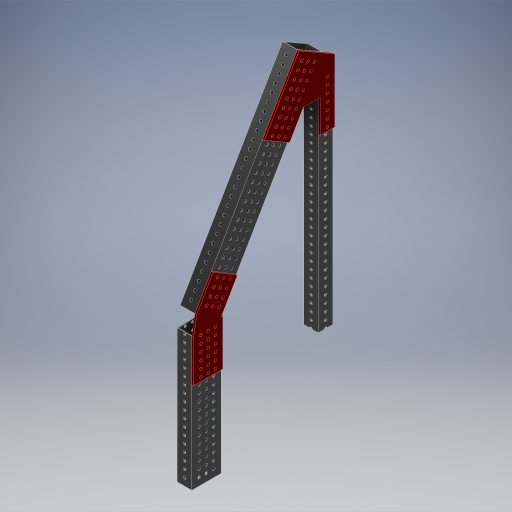
# Autodesk Inventor part: 2024-210-000-Fixed-Shootaur
Saved by Autodesk Inventor 2024.2 (Build 282272000, 272)
## iProperties
Created: 2024-01-23
Part Number: 2024-210-000-Fixed-Shootaur
Material: Generic
Document SubType Name: Modeling
Designer: rohan
Density: 1 g/cm^3
Appearance: Default
Author: rohan
Autodesk Inventor part; units mm, degrees
ref_plane "YZ Plane" through (0, 0, 0) normal (1, 0, 0) x (0, 1, 0)
ref_plane "XZ Plane" through (0, 0, 0) normal (0, 1, 0) x (-1, 0, 0)
ref_plane "XY Plane" through (0, 0, 0) normal (0, 0, 1) x (1, 0, 0)
sketch "Sketch1" plane through (0, 0, 0) normal (1, 0, 0) x (0, 1, 0)
  line L0 (47.3438, 284.2284) -> (278.9918, 284.2284)
  line L1 (278.9918, 284.2284) -> (278.9918, 233.4284)
  line L2 (278.9918, 233.4284) -> (47.3438, 233.4284)
  line L3 (618.5213, 101.1204) -> (593.1213, 57.1263)
  line L4 (593.1213, 57.1263) -> (285.1626, 234.9263)
  line L5 (285.1626, 234.9263) -> (310.5626, 278.9204)
  line L6 (310.5626, 278.9204) -> (618.5213, 101.1204)
  line L7 (285.1626, 234.9263) -> (285.1626, 48.2059)
  line L8 (310.5626, 278.9204) -> (324.8919, 270.6474)
  line L9 (47.3438, 233.4284) -> (47.3438, 284.2284)
  line L10 (47.3438, 284.2284) -> (21.9438, 284.2284)
  line L11 (21.9438, 284.2284) -> (21.9438, 233.4284)
  line L12 (21.9438, 233.4284) -> (47.3438, 233.4284)
  line L13 (47.3438, 233.4284) -> (47.3438, 284.2284)
  line L14 (21.9438, 64.4168) -> (72.7438, 64.4168)
  line L15 (72.7438, 64.4168) -> (72.7438, 39.0168)
  line L16 (72.7438, 39.0168) -> (21.9438, 39.0168)
  line L17 (21.9438, 39.0168) -> (21.9438, 64.4168)
  line L18 (21.9438, 284.2284) -> (72.7438, 284.2284)
  line L19 (72.7438, 284.2284) -> (72.7438, 724.8168)
  line L20 (72.7438, 724.8168) -> (21.9438, 724.8168)
  line L21 (21.9438, 724.8168) -> (21.9438, 284.2284)
  circle A0 centre (601.1727, 96.4718) radius 2.4892
  line L22 (72.7438, 64.4168) -> (123.5438, 64.4168)
  line L23 (123.5438, 64.4168) -> (123.5438, 39.0168)
  line L24 (123.5438, 39.0168) -> (72.7438, 39.0168)
  line L25 (72.7438, 39.0168) -> (72.7438, 64.4168)
  circle A1 centre (594.8227, 85.4733) radius 2.4892
  circle A2 centre (588.4727, 74.4748) radius 2.4892
  circle A3 centre (590.1742, 102.8218) radius 2.4892
  circle A4 centre (583.8242, 91.8233) radius 2.4892
  circle A5 centre (577.4742, 80.8248) radius 2.4892
  circle A6 centre (579.1757, 109.1718) radius 2.4892
  circle A7 centre (572.8257, 98.1733) radius 2.4892
  circle A8 centre (566.4757, 87.1748) radius 2.4892
  circle A9 centre (568.1772, 115.5218) radius 2.4892
  circle A10 centre (561.8272, 104.5233) radius 2.4892
  circle A11 centre (555.4772, 93.5248) radius 2.4892
  circle A12 centre (557.1787, 121.8718) radius 2.4892
  circle A13 centre (550.8287, 110.8733) radius 2.4892
  circle A14 centre (544.4787, 99.8748) radius 2.4892
  circle A15 centre (546.1801, 128.2218) radius 2.4892
  circle A16 centre (539.8301, 117.2233) radius 2.4892
  circle A17 centre (533.4801, 106.2248) radius 2.4892
  circle A18 centre (535.1816, 134.5718) radius 2.4892
  circle A19 centre (528.8316, 123.5733) radius 2.4892
  circle A20 centre (522.4816, 112.5748) radius 2.4892
  circle A21 centre (524.1831, 140.9218) radius 2.4892
  circle A22 centre (517.8331, 129.9233) radius 2.4892
  circle A23 centre (511.4831, 118.9248) radius 2.4892
  circle A24 centre (513.1846, 147.2718) radius 2.4892
  circle A25 centre (506.8346, 136.2733) radius 2.4892
  circle A26 centre (500.4846, 125.2748) radius 2.4892
  circle A27 centre (502.186, 153.6218) radius 2.4892
  circle A28 centre (495.836, 142.6233) radius 2.4892
  circle A29 centre (489.486, 131.6248) radius 2.4892
  circle A30 centre (491.1875, 159.9718) radius 2.4892
  circle A31 centre (484.8375, 148.9733) radius 2.4892
  circle A32 centre (478.4875, 137.9748) radius 2.4892
  circle A33 centre (480.189, 166.3218) radius 2.4892
  circle A34 centre (473.839, 155.3233) radius 2.4892
  circle A35 centre (467.489, 144.3248) radius 2.4892
  circle A36 centre (469.1905, 172.6718) radius 2.4892
  circle A37 centre (462.8405, 161.6733) radius 2.4892
  circle A38 centre (456.4905, 150.6748) radius 2.4892
  circle A39 centre (458.1919, 179.0218) radius 2.4892
  circle A40 centre (451.8419, 168.0233) radius 2.4892
  circle A41 centre (445.4919, 157.0248) radius 2.4892
  circle A42 centre (447.1934, 185.3718) radius 2.4892
  circle A43 centre (440.8434, 174.3733) radius 2.4892
  circle A44 centre (434.4934, 163.3748) radius 2.4892
  circle A45 centre (436.1949, 191.7218) radius 2.4892
  circle A46 centre (429.8449, 180.7233) radius 2.4892
  circle A47 centre (423.4949, 169.7248) radius 2.4892
  circle A48 centre (425.1964, 198.0718) radius 2.4892
  circle A49 centre (418.8464, 187.0733) radius 2.4892
  circle A50 centre (412.4964, 176.0748) radius 2.4892
  circle A51 centre (414.1979, 204.4218) radius 2.4892
  circle A52 centre (407.8479, 193.4233) radius 2.4892
  circle A53 centre (401.4979, 182.4248) radius 2.4892
  circle A54 centre (403.1993, 210.7718) radius 2.4892
  circle A55 centre (396.8493, 199.7733) radius 2.4892
  circle A56 centre (390.4993, 188.7748) radius 2.4892
  circle A57 centre (392.2008, 217.1218) radius 2.4892
  circle A58 centre (385.8508, 206.1233) radius 2.4892
  circle A59 centre (379.5008, 195.1248) radius 2.4892
  circle A60 centre (381.2023, 223.4718) radius 2.4892
  circle A61 centre (374.8523, 212.4733) radius 2.4892
  circle A62 centre (368.5023, 201.4748) radius 2.4892
  circle A63 centre (370.2038, 229.8218) radius 2.4892
  circle A64 centre (363.8538, 218.8233) radius 2.4892
  circle A65 centre (357.5038, 207.8248) radius 2.4892
  circle A66 centre (359.2052, 236.1718) radius 2.4892
  circle A67 centre (352.8552, 225.1733) radius 2.4892
  circle A68 centre (346.5052, 214.1748) radius 2.4892
  circle A69 centre (348.2067, 242.5218) radius 2.4892
  circle A70 centre (341.8567, 231.5233) radius 2.4892
  circle A71 centre (335.5067, 220.5248) radius 2.4892
  circle A72 centre (337.2082, 248.8718) radius 2.4892
  circle A73 centre (330.8582, 237.8733) radius 2.4892
  circle A74 centre (324.5082, 226.8748) radius 2.4892
  circle A75 centre (326.2097, 255.2218) radius 2.4892
  circle A76 centre (319.8597, 244.2233) radius 2.4892
  circle A77 centre (313.5097, 233.2248) radius 2.4892
  circle A78 centre (315.2112, 261.5718) radius 2.4892
  circle A79 centre (308.8612, 250.5733) radius 2.4892
  circle A80 centre (302.5112, 239.5748) radius 2.4892
  line L26 (123.5438, 64.4168) -> (568.0438, 64.4168)
  line L27 (568.0438, 64.4168) -> (568.0438, 39.0168)
  line L28 (568.0438, 39.0168) -> (123.5438, 39.0168)
  line L29 (123.5438, 39.0168) -> (123.5438, 64.4168)
  circle A81 centre (60.0438, 271.5284) radius 2.4892
  circle A82 centre (60.0438, 258.8284) radius 2.4892
  circle A83 centre (60.0438, 246.1284) radius 2.4892
  circle A84 centre (72.7438, 271.5284) radius 2.4892
  circle A85 centre (72.7438, 258.8284) radius 2.4892
  circle A86 centre (72.7438, 246.1284) radius 2.4892
  circle A87 centre (85.4438, 271.5284) radius 2.4892
  circle A88 centre (85.4438, 258.8284) radius 2.4892
  circle A89 centre (85.4438, 246.1284) radius 2.4892
  circle A90 centre (98.1438, 271.5284) radius 2.4892
  circle A91 centre (98.1438, 258.8284) radius 2.4892
  circle A92 centre (98.1438, 246.1284) radius 2.4892
  circle A93 centre (110.8438, 271.5284) radius 2.4892
  circle A94 centre (110.8438, 258.8284) radius 2.4892
  circle A95 centre (110.8438, 246.1284) radius 2.4892
  circle A96 centre (123.5438, 271.5284) radius 2.4892
  circle A97 centre (123.5438, 258.8284) radius 2.4892
  circle A98 centre (123.5438, 246.1284) radius 2.4892
  circle A99 centre (136.2438, 271.5284) radius 2.4892
  circle A100 centre (136.2438, 258.8284) radius 2.4892
  circle A101 centre (136.2438, 246.1284) radius 2.4892
  circle A102 centre (148.9438, 271.5284) radius 2.4892
  circle A103 centre (148.9438, 258.8284) radius 2.4892
  circle A104 centre (148.9438, 246.1284) radius 2.4892
  circle A105 centre (161.6438, 271.5284) radius 2.4892
  circle A106 centre (161.6438, 258.8284) radius 2.4892
  circle A107 centre (161.6438, 246.1284) radius 2.4892
  circle A108 centre (174.3438, 271.5284) radius 2.4892
  circle A109 centre (174.3438, 258.8284) radius 2.4892
  circle A110 centre (174.3438, 246.1284) radius 2.4892
  circle A111 centre (187.0438, 271.5284) radius 2.4892
  circle A112 centre (187.0438, 258.8284) radius 2.4892
  circle A113 centre (187.0438, 246.1284) radius 2.4892
  circle A114 centre (199.7438, 271.5284) radius 2.4892
  circle A115 centre (199.7438, 258.8284) radius 2.4892
  circle A116 centre (199.7438, 246.1284) radius 2.4892
  circle A117 centre (212.4438, 271.5284) radius 2.4892
  circle A118 centre (212.4438, 258.8284) radius 2.4892
  circle A119 centre (212.4438, 246.1284) radius 2.4892
  circle A120 centre (225.1438, 271.5284) radius 2.4892
  circle A121 centre (225.1438, 258.8284) radius 2.4892
  circle A122 centre (225.1438, 246.1284) radius 2.4892
  circle A123 centre (237.8438, 271.5284) radius 2.4892
  circle A124 centre (237.8438, 258.8284) radius 2.4892
  circle A125 centre (237.8438, 246.1284) radius 2.4892
  circle A126 centre (250.5438, 271.5284) radius 2.4892
  circle A127 centre (250.5438, 258.8284) radius 2.4892
  circle A128 centre (250.5438, 246.1284) radius 2.4892
  circle A129 centre (263.2438, 271.5284) radius 2.4892
  circle A130 centre (263.2438, 258.8284) radius 2.4892
  circle A131 centre (263.2438, 246.1284) radius 2.4892
  circle A132 centre (275.9438, 271.5284) radius 2.4892
  circle A133 centre (275.9438, 258.8284) radius 2.4892
  circle A134 centre (275.9438, 246.1284) radius 2.4892
  circle A135 centre (136.2438, 51.7168) radius 2.4892
  circle A136 centre (148.9438, 51.7168) radius 2.4892
  circle A137 centre (161.6438, 51.7168) radius 2.4892
  circle A138 centre (174.3438, 51.7168) radius 2.4892
  circle A139 centre (187.0438, 51.7168) radius 2.4892
  circle A140 centre (199.7438, 51.7168) radius 2.4892
  circle A141 centre (212.4438, 51.7168) radius 2.4892
  circle A142 centre (225.1438, 51.7168) radius 2.4892
  circle A143 centre (237.8438, 51.7168) radius 2.4892
  circle A144 centre (250.5438, 51.7168) radius 2.4892
  circle A145 centre (263.2438, 51.7168) radius 2.4892
  circle A146 centre (275.9438, 51.7168) radius 2.4892
  circle A147 centre (288.6438, 51.7168) radius 2.4892
  circle A148 centre (301.3438, 51.7168) radius 2.4892
  circle A149 centre (314.0438, 51.7168) radius 2.4892
  circle A150 centre (326.7438, 51.7168) radius 2.4892
  circle A151 centre (339.4438, 51.7168) radius 2.4892
  circle A152 centre (352.1438, 51.7168) radius 2.4892
  circle A153 centre (364.8438, 51.7168) radius 2.4892
  circle A154 centre (377.5438, 51.7168) radius 2.4892
  circle A155 centre (390.2438, 51.7168) radius 2.4892
  circle A156 centre (402.9438, 51.7168) radius 2.4892
  circle A157 centre (415.6438, 51.7168) radius 2.4892
  circle A158 centre (428.3438, 51.7168) radius 2.4892
  circle A159 centre (441.0438, 51.7168) radius 2.4892
  circle A160 centre (453.7438, 51.7168) radius 2.4892
  circle A161 centre (466.4438, 51.7168) radius 2.4892
  circle A162 centre (479.1438, 51.7168) radius 2.4892
  circle A163 centre (491.8438, 51.7168) radius 2.4892
  circle A164 centre (504.5438, 51.7168) radius 2.4892
  circle A165 centre (517.2438, 51.7168) radius 2.4892
  circle A166 centre (529.9438, 51.7168) radius 2.4892
  circle A167 centre (542.6438, 51.7168) radius 2.4892
  circle A168 centre (555.3438, 51.7168) radius 2.4892
  circle A169 centre (568.0438, 51.7168) radius 2.4892
  point P0 (72.7438, 51.7168)
  point P1 (568.0438, 49.2276)
  point P2 (568.0438, 54.206)
  dimension "d25" = 231.648
  dimension "d26" = 50.8
  dimension "d29" = 50.8
  dimension "d34" = 6.35
  dimension "d37" = 355.6
  dimension "d39" = 60
  dimension "d41" = 25.4
  dimension "d42" = 50.8
  dimension "d43" = 25.4
  dimension "d44" = 169.0116
  dimension "d45" = 50.8
  dimension "d46" = 440.5884
  dimension "d48" = 4.9784
  dimension "d59" = 50.8
  dimension "d60" = 12.7
  dimension "d61" = 12.7
  dimension "d64" = 12.7
  dimension "d67" = 12.7
  dimension "d70" = 444.5
  dimension "d87" = 4.9784
  dimension "d88" = 12.7
  dimension "d89" = 12.7
  dimension "d92" = 12.7
  dimension "d95" = 12.7
  dimension "d104" = 4.9784
  dimension "d105" = 12.7
  dimension "d106" = 12.7
  dimension "d109" = 12.7
  constraints: 170 centre point, 60 end point, 13 parallel, 8 horizontal, 8 perpendicular, 2 point on line, 2 vertical, 1 midpoint, 336 other
  measures "d25" distance of L1.end L2.end
  measures "d26" distance of L0.end L1.end
  measures "d29" distance of L3.start L3.end
  measures "d34" distance of L4.end L1.end
  measures "d37" distance between parallel lines of L5 L3
  measures "d39" angle of L4 L7
  measures "d41" distance of L12.end L11.end
  measures "d42" distance of L15.end L16.end
  measures "d43" distance of L14.end L15.end
  measures "d44" distance of L14.start L11.end
  measures "d45" distance of L20.end L19.end
  measures "d46" distance of L19.end L18.end
  measures "d48" diameter of A0
  measures "d59" distance of L23.end L24.end
  measures "d60" distance from line of L3 A0.centre
  measures "d61" distance from line of L6 A0.centre
  measures "d64" distance of A0.centre A1.centre
  measures "d67" distance of A0.centre A3.centre
  measures "d70" distance of L27.end L28.end
  measures "d87" diameter of A81
  measures "d88" distance from line of A81.centre L13
  measures "d89" distance from line of L18 A81.centre
  measures "d92" distance of A81.centre A82.centre
  measures "d95" distance of A81.centre A84.centre
  measures "d104" diameter of A135
  measures "d105" distance from line of L29 A135.centre
  measures "d106" distance from line of L26 A135.centre
  measures "d109" distance of A135.centre A136.centre
extrude "Extrusion1" add sketch "Sketch1" along normal blind 25.4 contours L3 L4 L5 L6
extrude "Extrusion2" add sketch "Sketch1" along normal blind 25.4 separate body contours L0 L1 L2 L9
extrude "Extrusion3" add sketch "Sketch1" along normal blind 25.4 separate body contours L26 L27 A169 L28 L23
sketch "Sketch2" plane through (0, 278.9918, 284.2284) normal (0, 1, 0) x (1, 0, 0)
  line L0 (0, 50.8) -> (0, 0) projected
  line L1 (0, 0) -> (25.4, 0) projected
  line L2 (25.4, 50.8) -> (25.4, 0) projected
  line L3 (0, 50.8) -> (25.4, 50.8) projected
  line L4 (23.8125, 1.5875) -> (1.5875, 1.5875)
  line L5 (1.5875, 1.5875) -> (1.5875, 49.2125)
  line L6 (1.5875, 49.2125) -> (23.8125, 49.2125)
  line L7 (23.8125, 49.2125) -> (23.8125, 1.5875)
  point P0 (0, 284.2284)
  dimension "d98" = 1.5875
  constraints: 8 end point, 3 other
  measures "d98" distance between parallel lines of L1 L4
extrude "Extrusion4" cut sketch "Sketch2" against normal blind 242.8875 contours L4 L5 L6 L7 bodies 2
sketch "Sketch3" plane through (0, 618.5213, 101.1204) normal (0, 0.8660254, -0.5) x (1, 0, 0)
  line L0 (0, 50.8) -> (0, 0) projected
  line L1 (0, 0) -> (25.4, 0) projected
  line L2 (25.4, 50.8) -> (25.4, 0) projected
  line L3 (0, 50.8) -> (25.4, 50.8) projected
  line L4 (23.8125, 1.5875) -> (1.5875, 1.5875)
  line L5 (1.5875, 1.5875) -> (1.5875, 49.2125)
  line L6 (1.5875, 49.2125) -> (23.8125, 49.2125)
  line L7 (23.8125, 49.2125) -> (23.8125, 1.5875)
  point P0 (0, 396.8334)
  dimension "d101" = 1.5875
  constraints: 8 end point, 3 other
  measures "d101" distance between parallel lines of L2 L7
extrude "Extrusion5" cut sketch "Sketch3" against normal up to surface (355.6 mm away) contours L4 L5 L6 L7 bodies 1
sketch "Sketch4" plane through (0, 123.5438, 39.0168) normal (0, -1, 0) x (1, 0, 0)
  line L0 (0, 25.4) -> (0, 0) projected
  line L1 (0, 0) -> (25.4, 0) projected
  line L2 (25.4, 25.4) -> (25.4, 0) projected
  line L3 (0, 25.4) -> (25.4, 25.4) projected
  line L4 (23.8125, 1.5875) -> (1.5875, 1.5875)
  line L5 (1.5875, 1.5875) -> (1.5875, 23.8125)
  line L6 (1.5875, 23.8125) -> (23.8125, 23.8125)
  line L7 (23.8125, 23.8125) -> (23.8125, 1.5875)
  point P0 (0, -39.0168)
  dimension "d114" = 1.5875
  constraints: 8 end point, 3 other
  measures "d114" distance between parallel lines of L2 L7
extrude "Extrusion6" cut sketch "Sketch4" against normal up to surface (444.5 mm away) contours L4 L5 L6 L7 bodies 3
sketch "Sketch5" plane through (25.4, 0, 0) normal (1, 0, 0) x (0, 0, -1)
  line L0 (-234.9263, 285.1626) -> (-57.1263, 593.1213) projected
  line L1 (-57.1263, 593.1213) -> (-101.1204, 618.5213) projected
  line L2 (-101.1204, 618.5213) -> (-278.9204, 310.5626) projected
  line L3 (-278.9204, 310.5626) -> (-234.9263, 285.1626) projected
  circle A0 centre (-239.5748, 302.5112) radius 2.4892 projected
  circle A1 centre (-250.5733, 308.8612) radius 2.4892 projected
  circle A2 centre (-261.5718, 315.2112) radius 2.4892 projected
  circle A3 centre (-233.2248, 313.5097) radius 2.4892 projected
  circle A4 centre (-244.2233, 319.8597) radius 2.4892 projected
  circle A5 centre (-255.2218, 326.2097) radius 2.4892 projected
  circle A6 centre (-226.8748, 324.5082) radius 2.4892 projected
  circle A7 centre (-237.8733, 330.8582) radius 2.4892 projected
  circle A8 centre (-248.8718, 337.2082) radius 2.4892 projected
  circle A9 centre (-220.5248, 335.5067) radius 2.4892 projected
  circle A10 centre (-231.5233, 341.8567) radius 2.4892 projected
  circle A11 centre (-242.5218, 348.2067) radius 2.4892 projected
  circle A12 centre (-214.1748, 346.5052) radius 2.4892 projected
  circle A13 centre (-225.1733, 352.8552) radius 2.4892 projected
  circle A14 centre (-236.1718, 359.2052) radius 2.4892 projected
  circle A15 centre (-207.8248, 357.5038) radius 2.4892 projected
  circle A16 centre (-218.8233, 363.8538) radius 2.4892 projected
  circle A17 centre (-229.8218, 370.2038) radius 2.4892 projected
  circle A18 centre (-201.4748, 368.5023) radius 2.4892 projected
  circle A19 centre (-212.4733, 374.8523) radius 2.4892 projected
  circle A20 centre (-223.4718, 381.2023) radius 2.4892 projected
  circle A21 centre (-195.1248, 379.5008) radius 2.4892 projected
  circle A22 centre (-206.1233, 385.8508) radius 2.4892 projected
  circle A23 centre (-217.1218, 392.2008) radius 2.4892 projected
  circle A24 centre (-188.7748, 390.4993) radius 2.4892 projected
  circle A25 centre (-199.7733, 396.8493) radius 2.4892 projected
  circle A26 centre (-210.7718, 403.1993) radius 2.4892 projected
  circle A27 centre (-182.4248, 401.4979) radius 2.4892 projected
  circle A28 centre (-193.4233, 407.8479) radius 2.4892 projected
  circle A29 centre (-204.4218, 414.1979) radius 2.4892 projected
  circle A30 centre (-176.0748, 412.4964) radius 2.4892 projected
  circle A31 centre (-187.0733, 418.8464) radius 2.4892 projected
  circle A32 centre (-198.0718, 425.1964) radius 2.4892 projected
  circle A33 centre (-169.7248, 423.4949) radius 2.4892 projected
  circle A34 centre (-180.7233, 429.8449) radius 2.4892 projected
  circle A35 centre (-191.7218, 436.1949) radius 2.4892 projected
  circle A36 centre (-163.3748, 434.4934) radius 2.4892 projected
  circle A37 centre (-174.3733, 440.8434) radius 2.4892 projected
  circle A38 centre (-185.3718, 447.1934) radius 2.4892 projected
  circle A39 centre (-157.0248, 445.4919) radius 2.4892 projected
  circle A40 centre (-168.0233, 451.8419) radius 2.4892 projected
  circle A41 centre (-179.0218, 458.1919) radius 2.4892 projected
  circle A42 centre (-150.6748, 456.4905) radius 2.4892 projected
  circle A43 centre (-161.6733, 462.8405) radius 2.4892 projected
  circle A44 centre (-172.6718, 469.1905) radius 2.4892 projected
  circle A45 centre (-144.3248, 467.489) radius 2.4892 projected
  circle A46 centre (-155.3233, 473.839) radius 2.4892 projected
  circle A47 centre (-166.3218, 480.189) radius 2.4892 projected
  circle A48 centre (-137.9748, 478.4875) radius 2.4892 projected
  circle A49 centre (-148.9733, 484.8375) radius 2.4892 projected
  circle A50 centre (-159.9718, 491.1875) radius 2.4892 projected
  circle A51 centre (-131.6248, 489.486) radius 2.4892 projected
  circle A52 centre (-142.6233, 495.836) radius 2.4892 projected
  circle A53 centre (-153.6218, 502.186) radius 2.4892 projected
  circle A54 centre (-125.2748, 500.4846) radius 2.4892 projected
  circle A55 centre (-136.2733, 506.8346) radius 2.4892 projected
  circle A56 centre (-147.2718, 513.1846) radius 2.4892 projected
  circle A57 centre (-118.9248, 511.4831) radius 2.4892 projected
  circle A58 centre (-129.9233, 517.8331) radius 2.4892 projected
  circle A59 centre (-140.9218, 524.1831) radius 2.4892 projected
  circle A60 centre (-112.5748, 522.4816) radius 2.4892 projected
  circle A61 centre (-123.5733, 528.8316) radius 2.4892 projected
  circle A62 centre (-134.5718, 535.1816) radius 2.4892 projected
  circle A63 centre (-106.2248, 533.4801) radius 2.4892 projected
  circle A64 centre (-117.2233, 539.8301) radius 2.4892 projected
  circle A65 centre (-128.2218, 546.1801) radius 2.4892 projected
  circle A66 centre (-99.8748, 544.4787) radius 2.4892 projected
  circle A67 centre (-110.8733, 550.8287) radius 2.4892 projected
  circle A68 centre (-121.8718, 557.1787) radius 2.4892 projected
  circle A69 centre (-93.5248, 555.4772) radius 2.4892 projected
  circle A70 centre (-104.5233, 561.8272) radius 2.4892 projected
  circle A71 centre (-115.5218, 568.1772) radius 2.4892 projected
  circle A72 centre (-87.1748, 566.4757) radius 2.4892 projected
  circle A73 centre (-98.1733, 572.8257) radius 2.4892 projected
  circle A74 centre (-109.1718, 579.1757) radius 2.4892 projected
  circle A75 centre (-80.8248, 577.4742) radius 2.4892 projected
  circle A76 centre (-91.8233, 583.8242) radius 2.4892 projected
  circle A77 centre (-102.8218, 590.1742) radius 2.4892 projected
  circle A78 centre (-74.4748, 588.4727) radius 2.4892 projected
  circle A79 centre (-85.4733, 594.8227) radius 2.4892 projected
  circle A80 centre (-96.4718, 601.1727) radius 2.4892 projected
  line L4 (-284.2284, 278.9918) -> (-284.2284, 47.3438) projected
  line L5 (-284.2284, 47.3438) -> (-233.4284, 47.3438) projected
  line L6 (-233.4284, 47.3438) -> (-233.4284, 278.9918) projected
  line L7 (-233.4284, 278.9918) -> (-284.2284, 278.9918) projected
  circle A81 centre (-246.1284, 275.9438) radius 2.4892 projected
  circle A82 centre (-271.5284, 275.9438) radius 2.4892 projected
  circle A83 centre (-258.8284, 263.2438) radius 2.4892 projected
  circle A84 centre (-246.1284, 250.5438) radius 2.4892 projected
  circle A85 centre (-271.5284, 250.5438) radius 2.4892 projected
  circle A86 centre (-258.8284, 237.8438) radius 2.4892 projected
  circle A87 centre (-246.1284, 225.1438) radius 2.4892 projected
  circle A88 centre (-271.5284, 225.1438) radius 2.4892 projected
  circle A89 centre (-258.8284, 212.4438) radius 2.4892 projected
  circle A90 centre (-246.1284, 199.7438) radius 2.4892 projected
  circle A91 centre (-271.5284, 199.7438) radius 2.4892 projected
  circle A92 centre (-258.8284, 187.0438) radius 2.4892 projected
  circle A93 centre (-246.1284, 174.3438) radius 2.4892 projected
  circle A94 centre (-271.5284, 174.3438) radius 2.4892 projected
  circle A95 centre (-258.8284, 161.6438) radius 2.4892 projected
  circle A96 centre (-246.1284, 148.9438) radius 2.4892 projected
  circle A97 centre (-271.5284, 148.9438) radius 2.4892 projected
  circle A98 centre (-258.8284, 136.2438) radius 2.4892 projected
  circle A99 centre (-246.1284, 123.5438) radius 2.4892 projected
  circle A100 centre (-271.5284, 123.5438) radius 2.4892 projected
  circle A101 centre (-258.8284, 110.8438) radius 2.4892 projected
  circle A102 centre (-246.1284, 98.1438) radius 2.4892 projected
  circle A103 centre (-271.5284, 98.1438) radius 2.4892 projected
  circle A104 centre (-258.8284, 85.4438) radius 2.4892 projected
  circle A105 centre (-246.1284, 72.7438) radius 2.4892 projected
  circle A106 centre (-271.5284, 72.7438) radius 2.4892 projected
  circle A107 centre (-258.8284, 60.0438) radius 2.4892 projected
  circle A108 centre (-271.5284, 60.0438) radius 2.4892 projected
  circle A109 centre (-246.1284, 60.0438) radius 2.4892 projected
  circle A110 centre (-258.8284, 72.7438) radius 2.4892 projected
  circle A111 centre (-271.5284, 85.4438) radius 2.4892 projected
  circle A112 centre (-246.1284, 85.4438) radius 2.4892 projected
  circle A113 centre (-258.8284, 98.1438) radius 2.4892 projected
  circle A114 centre (-271.5284, 110.8438) radius 2.4892 projected
  circle A115 centre (-246.1284, 110.8438) radius 2.4892 projected
  circle A116 centre (-258.8284, 123.5438) radius 2.4892 projected
  circle A117 centre (-271.5284, 136.2438) radius 2.4892 projected
  circle A118 centre (-246.1284, 136.2438) radius 2.4892 projected
  circle A119 centre (-258.8284, 148.9438) radius 2.4892 projected
  circle A120 centre (-271.5284, 161.6438) radius 2.4892 projected
  circle A121 centre (-246.1284, 161.6438) radius 2.4892 projected
  circle A122 centre (-258.8284, 174.3438) radius 2.4892 projected
  circle A123 centre (-271.5284, 187.0438) radius 2.4892 projected
  circle A124 centre (-246.1284, 187.0438) radius 2.4892 projected
  circle A125 centre (-258.8284, 199.7438) radius 2.4892 projected
  circle A126 centre (-271.5284, 212.4438) radius 2.4892 projected
  circle A127 centre (-246.1284, 212.4438) radius 2.4892 projected
  circle A128 centre (-258.8284, 225.1438) radius 2.4892 projected
  circle A129 centre (-271.5284, 237.8438) radius 2.4892 projected
  circle A130 centre (-246.1284, 237.8438) radius 2.4892 projected
  circle A131 centre (-258.8284, 250.5438) radius 2.4892 projected
  circle A132 centre (-271.5284, 263.2438) radius 2.4892 projected
  circle A133 centre (-246.1284, 263.2438) radius 2.4892 projected
  circle A134 centre (-258.8284, 275.9438) radius 2.4892 projected
  line L8 (-233.4284, 278.9918) -> (-233.4284, 206.0938)
  line L9 (-284.2284, 231.4938) -> (-284.2284, 278.9918)
  line L10 (-284.2284, 278.9918) -> (-278.9204, 310.5626)
  line L11 (-278.9204, 310.5626) -> (-250.3454, 360.056)
  line L12 (-250.3454, 360.056) -> (-206.911, 333.6864)
  line L13 (-233.4284, 278.9918) -> (-233.4284, 287.757)
  line L14 (-234.9263, 285.1626) -> (-57.1263, 593.1213) projected
  line L15 (-233.4284, 287.757) -> (-206.911, 333.6864)
  line L16 (-39.0168, 568.0438) -> (-49.2276, 568.0438) projected
  arc A135 (-54.206, 568.0438) -> (-49.2276, 568.0438) centre (-51.7168, 568.0438) ccw projected
  line L17 (-54.206, 568.0438) -> (-64.4168, 568.0438) projected
  line L18 (-64.4168, 568.0438) -> (-64.4168, 123.5438) projected
  line L19 (-64.4168, 123.5438) -> (-39.0168, 123.5438) projected
  line L20 (-39.0168, 123.5438) -> (-39.0168, 568.0438) projected
  circle A136 centre (-51.7168, 542.6438) radius 2.4892 projected
  circle A137 centre (-51.7168, 517.2438) radius 2.4892 projected
  circle A138 centre (-51.7168, 491.8438) radius 2.4892 projected
  circle A139 centre (-51.7168, 466.4438) radius 2.4892 projected
  circle A140 centre (-51.7168, 441.0438) radius 2.4892 projected
  circle A141 centre (-51.7168, 415.6438) radius 2.4892 projected
  circle A142 centre (-51.7168, 390.2438) radius 2.4892 projected
  circle A143 centre (-51.7168, 364.8438) radius 2.4892 projected
  circle A144 centre (-51.7168, 339.4438) radius 2.4892 projected
  circle A145 centre (-51.7168, 314.0438) radius 2.4892 projected
  circle A146 centre (-51.7168, 288.6438) radius 2.4892 projected
  circle A147 centre (-51.7168, 263.2438) radius 2.4892 projected
  circle A148 centre (-51.7168, 237.8438) radius 2.4892 projected
  circle A149 centre (-51.7168, 212.4438) radius 2.4892 projected
  circle A150 centre (-51.7168, 187.0438) radius 2.4892 projected
  circle A151 centre (-51.7168, 161.6438) radius 2.4892 projected
  circle A152 centre (-51.7168, 136.2438) radius 2.4892 projected
  circle A153 centre (-51.7168, 148.9438) radius 2.4892 projected
  circle A154 centre (-51.7168, 174.3438) radius 2.4892 projected
  circle A155 centre (-51.7168, 199.7438) radius 2.4892 projected
  circle A156 centre (-51.7168, 225.1438) radius 2.4892 projected
  circle A157 centre (-51.7168, 250.5438) radius 2.4892 projected
  circle A158 centre (-51.7168, 275.9438) radius 2.4892 projected
  circle A159 centre (-51.7168, 301.3438) radius 2.4892 projected
  circle A160 centre (-51.7168, 326.7438) radius 2.4892 projected
  circle A161 centre (-51.7168, 352.1438) radius 2.4892 projected
  circle A162 centre (-51.7168, 377.5438) radius 2.4892 projected
  circle A163 centre (-51.7168, 402.9438) radius 2.4892 projected
  circle A164 centre (-51.7168, 428.3438) radius 2.4892 projected
  circle A165 centre (-51.7168, 453.7438) radius 2.4892 projected
  circle A166 centre (-51.7168, 479.1438) radius 2.4892 projected
  circle A167 centre (-51.7168, 504.5438) radius 2.4892 projected
  circle A168 centre (-51.7168, 529.9438) radius 2.4892 projected
  circle A169 centre (-51.7168, 555.3438) radius 2.4892 projected
  line L21 (-101.1204, 618.5213) -> (-39.0168, 582.6658)
  line L22 (-39.0168, 582.6658) -> (-39.0168, 568.0438)
  line L23 (-39.0168, 568.0438) -> (-39.0168, 510.8938)
  line L24 (-39.0168, 510.8938) -> (-39.0168, 472.7938)
  line L25 (-39.0168, 472.7938) -> (-64.4168, 472.7938)
  line L26 (-64.4168, 472.7938) -> (-64.4168, 529.9438)
  line L27 (-101.1204, 618.5213) -> (-161.4454, 514.0353)
  line L28 (-101.1204, 618.5213) -> (-278.9204, 310.5626) projected
  line L29 (-161.4454, 514.0353) -> (-117.4513, 488.6353)
  line L30 (-64.4168, 529.9438) -> (-93.6018, 529.9438)
  line L31 (-117.4513, 488.6353) -> (-93.6018, 529.9438)
  line L32 (-58.5011, 593.915) -> (-236.3011, 285.9564) projected
  line L33 (-233.4284, 206.0938) -> (-284.2284, 206.0938)
  line L34 (-284.2284, 206.0938) -> (-284.2284, 231.4938)
  point P0 (0, 0)
  point P1 (-208.2684, 334.5105)
  dimension "d117" = 72.898
  dimension "d118" = 57.15
  dimension "d119" = 57.15
  dimension "d120" = 38.1
  dimension "d122" = 120.65
  constraints: 38 end point, 14 point on line, 4 collinear, 3 perpendicular, 1 horizontal, 1 parallel, 1 vertical
  measures "d117" distance of L6.end L8.end
  measures "d118" distance of L2.end L11.end
  measures "d119" distance of L16.start L23.end
  measures "d120" distance of L23.end L24.end
  measures "d122" distance of L1.end L27.end
extrude "Extrusion7" add sketch "Sketch5" along normal blind 3.175 separate body contours L0 L13 L7 L10 L3 | L3 L2 L12 L32 | L6 L33 L4 L7
extrude "Extrusion8" add sketch "Sketch5" along normal blind 3.175 separate body contours L29 L32 L1 L0 | L29 L2 L1 L32 | L0 L21 L22 L16 A135 L17 L18 L30 | L18 L17 A135 L16 L20 L25
sketch "Sketch6" plane through (0, 123.5438, 39.0168) normal (0, 0, -1) x (-1, 0, 0)
  line L0 (0, 0) -> (0, 444.5) projected
  line L1 (0, 444.5) -> (-25.4, 444.5) projected
  line L2 (-25.4, 0) -> (-25.4, 444.5) projected
  line L3 (0, 0) -> (-25.4, 0) projected
  circle A0 centre (-12.7, 12.7) radius 2.4892
  circle A1 centre (-12.7, 25.4) radius 2.4892
  circle A2 centre (-12.7, 38.1) radius 2.4892
  circle A3 centre (-12.7, 50.8) radius 2.4892
  circle A4 centre (-12.7, 63.5) radius 2.4892
  circle A5 centre (-12.7, 76.2) radius 2.4892
  circle A6 centre (-12.7, 88.9) radius 2.4892
  circle A7 centre (-12.7, 101.6) radius 2.4892
  circle A8 centre (-12.7, 114.3) radius 2.4892
  circle A9 centre (-12.7, 127) radius 2.4892
  circle A10 centre (-12.7, 139.7) radius 2.4892
  circle A11 centre (-12.7, 152.4) radius 2.4892
  circle A12 centre (-12.7, 165.1) radius 2.4892
  circle A13 centre (-12.7, 177.8) radius 2.4892
  circle A14 centre (-12.7, 190.5) radius 2.4892
  circle A15 centre (-12.7, 203.2) radius 2.4892
  circle A16 centre (-12.7, 215.9) radius 2.4892
  circle A17 centre (-12.7, 228.6) radius 2.4892
  circle A18 centre (-12.7, 241.3) radius 2.4892
  circle A19 centre (-12.7, 254) radius 2.4892
  circle A20 centre (-12.7, 266.7) radius 2.4892
  circle A21 centre (-12.7, 279.4) radius 2.4892
  circle A22 centre (-12.7, 292.1) radius 2.4892
  circle A23 centre (-12.7, 304.8) radius 2.4892
  circle A24 centre (-12.7, 317.5) radius 2.4892
  circle A25 centre (-12.7, 330.2) radius 2.4892
  circle A26 centre (-12.7, 342.9) radius 2.4892
  circle A27 centre (-12.7, 355.6) radius 2.4892
  circle A28 centre (-12.7, 368.3) radius 2.4892
  circle A29 centre (-12.7, 381) radius 2.4892
  circle A30 centre (-12.7, 393.7) radius 2.4892
  circle A31 centre (-12.7, 406.4) radius 2.4892
  circle A32 centre (-12.7, 419.1) radius 2.4892
  circle A33 centre (-12.7, 431.8) radius 2.4892
  circle A34 centre (-12.7, 444.5) radius 2.4892
  point P0 (0, -123.5438)
  point P1 (-12.7, 444.5)
  point P2 (-15.1892, 444.5)
  point P3 (-10.2108, 444.5)
  dimension "d130" = 4.9784
  dimension "d131" = 12.7
  dimension "d132" = 12.7
  dimension "d135" = 12.7
  constraints: 35 centre point, 1 midpoint, 1 vertical, 68 other
  measures "d130" diameter of A0
  measures "d131" distance from line of A0.centre L3
  measures "d132" distance from line of L0 A0.centre
  measures "d135" distance of A0.centre A1.centre
extrude "Extrusion9" cut sketch "Sketch6" against normal up to surface (25.4 mm away) contours A34 L1 | A0 | A1 | A2 | A3 | A4 | A5 | A6 | A7 | A8 | A9 | A10 | A11 | A12 | A13 | A14 | A15 | A16 | A17 | A18 | A19 | A20 | A21 | A22 | A23 | A24 | A25 | A26 | A27 | A28 | A29 | A30 | A31 | A32 | A33 picked at (-12.4058, 442.953) bodies 3
sketch "Sketch7" plane through (0, 310.5626, 278.9204) normal (0, 0.5, 0.8660254) x (1, 0, 0)
  line L0 (0, 355.6) -> (0, 0) projected
  line L1 (0, 0) -> (25.4, 0) projected
  line L2 (25.4, 355.6) -> (25.4, 0) projected
  line L3 (0, 355.6) -> (25.4, 355.6) projected
  circle A0 centre (12.7, 342.9) radius 2.4892
  circle A1 centre (12.7, 330.2) radius 2.4892
  circle A2 centre (12.7, 317.5) radius 2.4892
  circle A3 centre (12.7, 304.8) radius 2.4892
  circle A4 centre (12.7, 292.1) radius 2.4892
  circle A5 centre (12.7, 279.4) radius 2.4892
  circle A6 centre (12.7, 266.7) radius 2.4892
  circle A7 centre (12.7, 254) radius 2.4892
  circle A8 centre (12.7, 241.3) radius 2.4892
  circle A9 centre (12.7, 228.6) radius 2.4892
  circle A10 centre (12.7, 215.9) radius 2.4892
  circle A11 centre (12.7, 203.2) radius 2.4892
  circle A12 centre (12.7, 190.5) radius 2.4892
  circle A13 centre (12.7, 177.8) radius 2.4892
  circle A14 centre (12.7, 165.1) radius 2.4892
  circle A15 centre (12.7, 152.4) radius 2.4892
  circle A16 centre (12.7, 139.7) radius 2.4892
  circle A17 centre (12.7, 127) radius 2.4892
  circle A18 centre (12.7, 114.3) radius 2.4892
  circle A19 centre (12.7, 101.6) radius 2.4892
  circle A20 centre (12.7, 88.9) radius 2.4892
  circle A21 centre (12.7, 76.2) radius 2.4892
  circle A22 centre (12.7, 63.5) radius 2.4892
  circle A23 centre (12.7, 50.8) radius 2.4892
  circle A24 centre (12.7, 38.1) radius 2.4892
  circle A25 centre (12.7, 25.4) radius 2.4892
  circle A26 centre (12.7, 12.7) radius 2.4892
  point P0 (0, -129.4949)
  point P1 (12.7, 355.6)
  dimension "d142" = 4.9784
  dimension "d143" = 12.7
  dimension "d144" = 12.7
  dimension "d147" = 12.7
  constraints: 27 centre point, 1 midpoint, 1 vertical, 52 other
  measures "d142" diameter of A0
  measures "d143" distance of point (12.7, 355.6) A0.centre
  measures "d144" distance from line of L0 A0.centre
  measures "d147" distance of A0.centre A1.centre
extrude "Extrusion10" cut sketch "Sketch7" against normal up to surface (50.8 mm away) contours A0 | A1 | A2 | A3 | A4 | A5 | A6 | A7 | A8 | A9 | A10 | A11 | A12 | A13 | A14 | A15 | A16 | A17 | A18 | A19 | A20 | A21 | A22 | A23 | A24 | A25 | A26 bodies 1
sketch "Sketch8" plane through (0, 47.3438, 284.2284) normal (0, 0, 1) x (1, 0, 0)
  line L0 (0, 231.648) -> (0, 0) projected
  line L1 (0, 0) -> (25.4, 0) projected
  line L2 (25.4, 231.648) -> (25.4, 0) projected
  line L3 (0, 231.648) -> (25.4, 231.648) projected
  circle A0 centre (12.7, 12.7) radius 2.4892
  circle A1 centre (12.7, 25.4) radius 2.4892
  circle A2 centre (12.7, 38.1) radius 2.4892
  circle A3 centre (12.7, 50.8) radius 2.4892
  circle A4 centre (12.7, 63.5) radius 2.4892
  circle A5 centre (12.7, 76.2) radius 2.4892
  circle A6 centre (12.7, 88.9) radius 2.4892
  circle A7 centre (12.7, 101.6) radius 2.4892
  circle A8 centre (12.7, 114.3) radius 2.4892
  circle A9 centre (12.7, 127) radius 2.4892
  circle A10 centre (12.7, 139.7) radius 2.4892
  circle A11 centre (12.7, 152.4) radius 2.4892
  circle A12 centre (12.7, 165.1) radius 2.4892
  circle A13 centre (12.7, 177.8) radius 2.4892
  circle A14 centre (12.7, 190.5) radius 2.4892
  circle A15 centre (12.7, 203.2) radius 2.4892
  circle A16 centre (12.7, 215.9) radius 2.4892
  circle A17 centre (12.7, 228.6) radius 2.4892
  point P0 (0, -47.3438)
  point P1 (12.7, 231.648)
  point P2 (12.7, 0)
  dimension "d166" = 4.9784
  dimension "d167" = 12.7
  dimension "d168" = 12.7
  dimension "d171" = 12.7
  constraints: 18 centre point, 2 midpoint, 1 vertical, 34 other
  measures "d166" diameter of A0
  measures "d167" distance of A0.centre point (12.7, 0)
  measures "d168" distance from line of L2 A0.centre
  measures "d171" distance of A0.centre A1.centre
extrude "Extrusion12" cut sketch "Sketch8" against normal up to surface (50.8 mm away) contours A0 | A1 | A2 | A3 | A4 | A5 | A6 | A7 | A8 | A9 | A10 | A11 | A12 | A13 | A14 | A15 | A16 | A17 bodies 2
sketch "Sketch9" plane through (0, 123.5438, 39.0168) normal (0, -1, 0) x (1, 0, 0)
  line L0 (23.8125, 23.8125) -> (23.8125, 1.5875) projected
  line L1 (23.8125, 1.5875) -> (1.5875, 1.5875) projected
  line L2 (1.5875, 1.5875) -> (1.5875, 23.8125) projected
  line L3 (1.5875, 23.8125) -> (23.8125, 23.8125) projected
  line L4 (0, 25.4) -> (0, 0) projected
  line L5 (0, 0) -> (25.4, 0) projected
  line L6 (25.4, 25.4) -> (25.4, 0) projected
  line L7 (0, 25.4) -> (25.4, 25.4) projected
  point P0 (0, -39.0168)
extrude "Extrusion13" cut sketch "Sketch9" against normal blind 50.8 bodies 3
